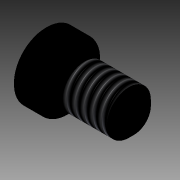
# Autodesk Inventor part: 2750-0.250
Saved by Autodesk Inventor 2014 SP2 (Build 180246200, 246)
## iProperties
Created: 2019-11-08
Part Number: 2750-0.250
Material: Generic
Catalog Web Link: www.cadenas.de
Description: 2750_bolt-Socket Head Cap Screws
Vendor: 8020
Document SubType Name: Modeling
Designer: psadmin
Manufacturer: 8020
Mass: 0.508924 g
Surface Area: 4.31943 cm^2
Volume: 0.508924 cm^3
Density: 1 g/cm^3
Appearance: PSOLRGB-0-0-0
Category: PARTsolutions
Company: 8020
Title: 2750-0.250
Author: Cadenas PARTsolutions
Comments: Socket Head Cap Screws
PSOL_IDENT_0: {$CADENAS_DATA\23d-libs\8020\inch\linear_motion\2750_bolt.prj},163 {VTYP=3D},{NB=2750-0.250},{LINA=2
PSOL_IDENT_1: 750-0.250},{NN=2750_bolt},{DATE=01.10.2019 06:04:24},{GEOMDATE=12.03.2012 09:23:00},{VERSION=},{LINE
PSOL_IDENT_2: ID=60},{WBVAR=},{WBNUMERIC=}  {NB=2750-0.250},{LINA=2750-0.250},{KT=DUMMY},{PN=2750-0.250},{THRD=1/4
PSOL_IDENT_3: -20},{THRD1=0.2500},{FIN=Black Zinc},{L=0.375},{TT=UNC},{A=0.375},{H=0.127},{J=0.12500},{T=0.064},{T
PSOL_IDENT_4: H=0.2500},{NT=3204}
NN: 2750_bolt
NT: 3204
NB: 2750-0.250
NBSYN: $PN.
LINA: 2750-0.250
PN: 2750-0.250
THRD: 1/4-20
FIN: Black Zinc
L: 0.375
A: 0.375
H: 0.127
J: 0.125
SUPPLIER: 8020
ARTICLENO: 2750-0.250
BOMINFO: 2750-0.250
CREATOR: CADENAS GmbH
Autodesk Inventor part; units mm, degrees
sketch "Sketch_1" plane through (0, 0, 0) normal (0, 0, 1) x (1, 0, 0)
  line L0 (9.525, 0) -> (-3.2258, 0)
  line L1 (-3.2258, 0) -> (-3.2258, 4.6101)
  line L2 (-3.2258, 4.6101) -> (-3.0734, 4.7625)
  line L3 (-3.0734, 4.7625) -> (-0.254, 4.7625)
  arc A0 (0, 4.5085) -> (-0.254, 4.7625) centre (-0.254, 4.5085) ccw
  line L4 (0, 4.5085) -> (0, 3.2512)
  arc A1 (0, 3.2512) -> (0.0762, 3.175) centre (0.0762, 3.2512) ccw
  line L5 (0.0762, 3.175) -> (8.7693, 3.175)
  line L6 (8.7693, 3.175) -> (9.525, 2.4194)
  line L7 (9.525, 2.4194) -> (9.525, 0)
  line L8 (9.525, 0) -> (-3.2258, 0)
  constraints: 18 end point, 4 point on circle, 2 centre point
revolve "Revolution1" add sketch "Sketch_1" angle 360 about axis through (9.525, 0, 0) along (1, 0, 0)
thread "Thread1" size "1/4-20 UNC" class "2A" standard "ANSI Unified Screw Threads" length 6.3881
sketch "Sketch_3" plane through (-3.2258, 0, 0) normal (1, 0, 0) x (0, 0, -1)
  line L0 (-1.5875, -0.9165) -> (0, -1.8331)
  line L1 (0, -1.8331) -> (1.5875, -0.9165)
  line L2 (1.5875, -0.9165) -> (1.5875, 0.9165)
  line L3 (1.5875, 0.9165) -> (0, 1.8331)
  line L4 (0, 1.8331) -> (-1.5875, 0.9165)
  line L5 (-1.5875, 0.9165) -> (-1.5875, -0.9165)
  constraints: 12 end point
extrude "Extrusion1" cut sketch "Sketch_3" along normal blind 1.6256
sketch "Sketch_4" plane through (0, 0, 0) normal (0, 0, 1) x (1, 0, 0)
  line L0 (-0.6837, 0) -> (-1.6002, 0)
  line L1 (-1.6002, 0) -> (-1.6002, 1.5875)
  line L2 (-1.6002, 1.5875) -> (-0.6837, 0)
  line L3 (-0.6837, 0) -> (-1.6002, 0)
  constraints: 8 end point
revolve "Revolution2" cut sketch "Sketch_4" angle 360 about axis through (-0.6837, 0, 0) along (1, 0, 0)
ref_plane "screw_XY" through (0, 0, 0) normal (1, 0, 0) x (0, 0, -1)
ref_plane "screw_YZ" through (0, 0, 0) normal (0, 0, -1) x (0, 1, 0)
ref_plane "screw_ZX" through (0, 0, 0) normal (0, 1, 0) x (1, 0, 0)
ref_plane "screw1_XY" through (9.525, 0, 0) normal (1, 0, 0) x (0, 0, -1)
ref_plane "screw1_YZ" through (9.525, 0, 0) normal (0, 0, -1) x (0, 1, 0)
ref_plane "screw1_ZX" through (9.525, 0, 0) normal (0, 1, 0) x (1, 0, 0)
ref_plane "screw2_XY" through (4.445, 0, 0) normal (1, 0, 0) x (0, 0, -1)
ref_plane "screw2_YZ" through (4.445, 0, 0) normal (0, 0, -1) x (0, 1, 0)
ref_plane "screw2_ZX" through (4.445, 0, 0) normal (0, 1, 0) x (1, 0, 0)
ref_plane "to_tnut_XY" through (7.366, 0, 0) normal (1, 0, 0) x (0, 0, -1)
ref_plane "to_tnut_YZ" through (7.366, 0, 0) normal (0, 0, -1) x (0, 1, 0)
ref_plane "to_tnut_ZX" through (7.366, 0, 0) normal (0, 1, 0) x (1, 0, 0)
body "Solid1"
